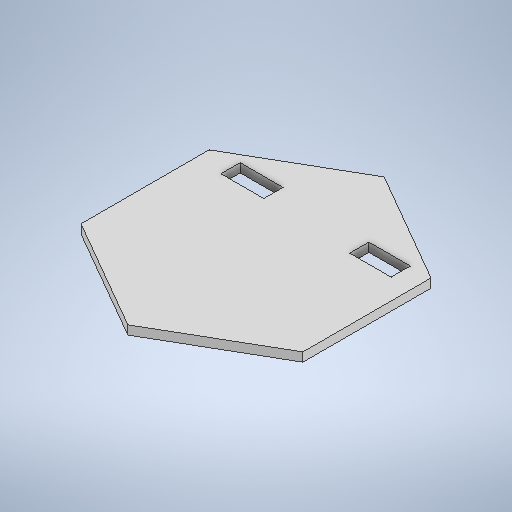
# Autodesk Inventor part: baseBody
Saved by Autodesk Inventor 2025.1 (Build 291241020, 241B)
## iProperties
Created: 2025-03-08
Part Number: baseBody
Material: Generic
Document SubType Name: Modeling
Designer: omiye
Density: 1 g/cm^3
Appearance: Default
Author: omiye
Autodesk Inventor part; units mm, degrees
ref_plane "YZ Plane" through (0, 0, 0) normal (1, 0, 0) x (0, 1, 0)
ref_plane "XZ Plane" through (0, 0, 0) normal (0, 1, 0) x (-1, 0, 0)
ref_plane "XY Plane" through (0, 0, 0) normal (0, 0, 1) x (1, 0, 0)
sketch "Sketch1" plane through (0, 0, 0) normal (0, 1, 0) x (-1, 0, 0)
  line L0 (0, 0) -> (75, 0)
  line L1 (0, 0) -> (75, 0) construction
  line L2 (75, -43.3013) -> (0, -86.6025)
  line L3 (0, -86.6025) -> (-75, -43.3013)
  line L4 (-75, -43.3013) -> (-75, 43.3013)
  line L5 (-75, 43.3013) -> (0, 86.6025)
  line L6 (0, 86.6025) -> (75, 43.3013)
  line L7 (75, 43.3013) -> (75, -43.3013)
  dimension "d0" = 75
  dimension "d1" = 0
  constraints: 16 end point, 2 horizontal, 1 coincident, 1 collinear, 1 midpoint, 13 other
  measures "d0" distance of L0.start L0.end
  measures "d1" distance between parallel lines of L0 L1
extrude "Extrusion1" add sketch "Sketch1" along normal blind 6
sketch "Sketch9" plane through (0, 6, 0) normal (0, 1, 0) x (1, 0, 0)
  line L0 (-75, 43.3013) -> (-75, -43.3013) projected
  line L1 (-75, 43.3013) -> (-50, 43.3013)
  line L2 (75, 43.3013) -> (0, 86.6025) projected
  line L3 (75, 43.3013) -> (55, 43.3013)
  line L4 (55, 43.3013) -> (55, 30.3013)
  line L5 (55, 30.3013) -> (33, 30.3013)
  line L6 (33, 30.3013) -> (33, 43.3013)
  line L7 (33, 43.3013) -> (55, 43.3013)
  line L8 (-50, 43.3013) -> (-50, 33.3013)
  line L9 (-50, 33.3013) -> (-28, 33.3013)
  line L10 (-28, 33.3013) -> (-28, 43.3013)
  line L11 (-28, 43.3013) -> (-50, 43.3013)
  line L12 (-28, 43.3013) -> (-50, 43.3013)
  line L13 (-50, 43.3013) -> (-50, 46.3013)
  line L14 (-50, 46.3013) -> (-28, 46.3013)
  line L15 (-28, 46.3013) -> (-28, 43.3013)
  line L16 (-50, 33.3013) -> (-50, 46.3013)
  line L17 (-50, 46.3013) -> (-57, 46.3013)
  line L18 (-57, 46.3013) -> (-57, 33.3013)
  line L19 (-57, 33.3013) -> (-50, 33.3013)
  line L20 (55, 43.3013) -> (55, 30.3013)
  line L21 (55, 30.3013) -> (61, 30.3013)
  line L22 (61, 30.3013) -> (61, 43.3013)
  line L23 (61, 43.3013) -> (55, 43.3013)
  point P0 (0, 0)
  dimension "d26" = 25
  dimension "d27" = 20
  dimension "d28" = 13
  dimension "d29" = 22
  dimension "d30" = 10
  dimension "d31" = 22
  dimension "d32" = 3
  dimension "d33" = 7
  dimension "d34" = 6
  constraints: 44 end point, 10 parallel, 6 perpendicular, 3 collinear, 2 horizontal, 1 vertical
  measures "d26" distance of L0.start L1.end
  measures "d27" distance of L2.start L3.end
  measures "d28" distance of L3.end L4.end
  measures "d29" distance of L4.end L5.end
  measures "d30" distance of L1.end L8.end
  measures "d31" distance of L9.end L8.end
  measures "d32" distance of L1.end L13.end
  measures "d33" distance of L17.end L13.end
  measures "d34" distance of L21.end L4.end
extrude "Extrusion2" cut sketch "Sketch9" against normal blind 10
body "Solid1"
